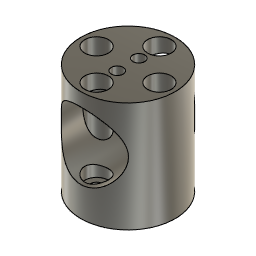
17mm-marker-holder v2 (Autodesk Fusion 360 design; units mm, degrees)
Autodesk Fusion 360 part; units mm, degrees
note: some values were not read from the file. Set by a fixed rule: which sketch regions a step uses.
sketch "Sketch1" plane through (0, 0, 0) normal (0, 0, 1) x (1, 0, 0)
  circle A0 centre (-8, 0) radius 1.5
  circle A1 centre (8, 0) radius 1.5
  circle A2 centre (0, -8) radius 1.5
  circle A3 centre (0, 8) radius 1.5
  circle A4 centre (0, 0) radius 12
  dimension "d3" = 3
  dimension "d4" = 8
  dimension "d5" = 3
  dimension "d6" = 3
  dimension "d7" = 3
  dimension "d8" = 8
  dimension "d9" = 8
  dimension "d10" = 8
  dimension "d19" = 24
  constraint coincident A4.centre origin
  measures "d3" diameter of A0
  measures "d4" distance of A4.centre A0.centre
  measures "d5" diameter of A1
  measures "d6" diameter of A2
  measures "d7" diameter of A3
  measures "d8" distance of A4.centre A2.centre
  measures "d9" distance of A4.centre A3.centre
  measures "d10" distance of A4.centre A1.centre
  measures "d19" diameter of A4
extrude "Extrude1" add sketch "Sketch1" along normal blind 20
extrude "Extrude2" cut 1 faces at (0.0374, 2.1681, 20) along direction (0, 0, -1) blind 12
sketch "Sketch2" plane through (0, 0, 8) normal (0, 0, 1) x (-1, 0, 0)
  circle A0 centre (0, -8) radius 1.5
  circle A1 centre (-8, 0) radius 1.5
  circle A2 centre (0, 8) radius 1.5
  circle A3 centre (8, 0) radius 1.5
  circle A4 centre (0, -8) radius 3
  circle A5 centre (8, 0) radius 3
  circle A6 centre (-8, 0) radius 3
  circle A7 centre (0, 8) radius 3
  circle A8 centre (0, 0) radius 12
  dimension "d15" = 6
  constraint concentric A0 A4
  constraint concentric A3 A5
  constraint concentric A1 A6
  constraint concentric A2 A7
  measures "d15" diameter of A4
extrude "Extrude3" cut sketch "Sketch2" against normal blind 3 contours A4
extrude "Extrude4" cut sketch "Sketch2" against normal blind 3 contours A5
extrude "Extrude5" cut sketch "Sketch2" against normal blind 3 contours A7
extrude "Extrude6" cut sketch "Sketch2" against normal blind 3 contours A6
extrude "Extrude7" add 1 faces at (-0.0747, -1.6695, 8) along direction (0, 0, 1) blind 20
hole "Hole1" at (0, -12, 16.0718) direction (0, 1, 0) diameter 17.1 depth 25 tip angle 180
sketch "Sketch3" plane through (0, 0, 28) normal (0, 0, 1) x (-1, 0, 0)
  circle A0 centre (-8, 0) radius 3
  circle A1 centre (0, 8) radius 3
  circle A2 centre (8, 0) radius 3
  circle A3 centre (0, -8) radius 3
  circle A4 centre (0, 0) radius 12
  circle A5 centre (0, -2.75) radius 1.5
  circle A6 centre (0, 2.75) radius 1.5
  circle A7 centre (0, 2.75) radius 2.5
  circle A8 centre (0, -2.75) radius 2.5
  dimension "d31" = 3
  dimension "d32" = 3
  dimension "d33" = 2.75
  dimension "d34" = 2.75
  dimension "d39" = 5
  dimension "d40" = 5
  constraint concentric A6 A7
  constraint concentric A5 A8
  measures "d31" diameter of A5
  measures "d32" diameter of A6
  measures "d33" distance of A4.centre A5.centre
  measures "d34" distance of A4.centre A6.centre
  measures "d39" diameter of A7
  measures "d40" diameter of A8
extrude "Extrude8" cut sketch "Sketch3" against normal blind 5 contours A5
extrude "Extrude9" cut sketch "Sketch3" against normal blind 5 contours A6
